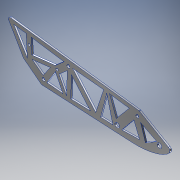
# Autodesk Inventor part: bracket1
Saved by Autodesk Inventor 2018.2 (Build 222227000, 227)
## iProperties
Created: 2018-03-05
Part Number: bracket1
Material: アルミニウム 6061
Document SubType Name: Modeling
Designer: ku_sk
Density: 2.7 g/cm^3
Appearance: アルミニウム - フラット
Mass: 349.891 g
Surface Area: 692.084 cm^2
Volume: 129.589 cm^3
Author: ku_sk
Autodesk Inventor part; units mm, degrees
ref_plane "YZ Plane" through (0, 0, 0) normal (1, 0, 0) x (0, 1, 0)
ref_plane "XZ Plane" through (0, 0, 0) normal (0, 1, 0) x (-1, 0, 0)
ref_plane "XY Plane" through (0, 0, 0) normal (0, 0, 1) x (1, 0, 0)
sketch "スケッチ2" plane through (0, 0, 0) normal (0, 1, 0) x (-1, 0, 0)
  arc A0 (320.7468, 34.8983) -> (392.1215, 71.6787) centre (243.1623, 273.099) ccw projected
  arc A1 (310.5095, 31.8959) -> (320.7468, 34.8983) centre (264.9264, 206.2785) ccw projected
  arc A2 (290.9118, 29.5172) -> (310.5095, 31.8959) centre (291.9468, 102.9093) ccw projected
  arc A3 (278.6891, 31.4878) -> (290.9118, 29.5172) centre (291.5128, 72.1352) ccw projected
  arc A4 (274.9831, 33.389) -> (278.6891, 31.4878) centre (282.4278, 43.3382) ccw projected
  arc A5 (275.4733, 39.2078) -> (274.9831, 33.389) centre (277.0456, 36.1453) ccw projected
  arc A6 (283.1253, 42.3274) -> (275.4733, 39.2078) centre (297.1464, -3.0086) ccw projected
  arc A7 (310.1184, 49.282) -> (283.1253, 42.3274) centre (369.3413, -236.446) ccw projected
  arc A8 (310.1184, 49.282) -> (326.9533, 52.7997) centre (-771.7798, 5269.0252) ccw projected
  arc A9 (326.9533, 52.7997) -> (357.98, 60.8795) centre (256.8539, 385.5961) ccw projected
  arc A10 (357.98, 60.8795) -> (391.1188, 73.3957) centre (268.9975, 346.6028) ccw projected
  arc A11 (392.1215, 71.6787) -> (391.1188, 73.3957) centre (391.5269, 72.4828) ccw projected
  circle A12 centre (287.1934, 37.1564) radius 3 projected
  circle A13 centre (359.7933, 56.2153) radius 3 projected
  arc A14 (100.5026, -29.4375) -> (303.8176, 17.6729) centre (68.6386, 570.3585) ccw projected
  arc A15 (74.9408, -30.0377) -> (100.5026, -29.4375) centre (77.5861, 401.9345) ccw projected
  arc A16 (28.1912, -23.4013) -> (74.9408, -30.0377) centre (76.0159, 145.5175) ccw projected
  arc A17 (1.2395, -11.312) -> (28.1912, -23.4013) centre (55.8939, 74.446) ccw projected
  arc A18 (-6.0217, -4.7376) -> (1.2395, -11.312) centre (16.9451, 13.3315) ccw projected
  arc A19 (-1.6159, 7.4897) -> (-6.0217, -4.7376) centre (0, 0) ccw projected
  arc A20 (17.9572, 9.9554) -> (-1.6159, 7.4897) centre (22.277, -103.2534) ccw projected
  arc A21 (84.7958, 9.311) -> (17.9572, 9.9554) centre (44.6377, -689.2581) ccw projected
  arc A22 (84.7958, 9.311) -> (126.0099, 7.0084) centre (819.0754, 12782.4716) ccw projected
  arc A23 (126.0099, 7.0084) -> (203.0122, 6.466) centre (170.258, 822.6468) ccw projected
  arc A24 (203.0122, 6.466) -> (303.8176, 17.6729) centre (174.1884, 724.7085) ccw projected
  circle A25 centre (20.0666, -1.5588) radius 5 projected
  circle A26 centre (130.4331, -10.1322) radius 5 projected
  line L0 (100.5026, -29.4375) -> (327.9026, -17.3569)
  line L1 (-3.831, 6.6355) -> (72.6844, 50.8117)
  line L2 (1137.2465, 0) -> (-1089.9509, 0) projected
  line L3 (72.6844, 50.8117) -> (483.7253, 102.9093)
  line L4 (327.9026, -17.3569) -> (483.7253, 102.9093)
  point P0 (0, 0)
  point P1 (371.2778, 57.8193)
  dimension "d7" = 30
  constraints: 8 end point, 2 point on circle, 2 tangent
  measures "d7" angle of L2 L1
extrude "押し出し3" add sketch "スケッチ2" along normal blind 4 contours A1 A2 A3 A4 A5 A6 A7 A8 A9 A10 A11 A0 | A15 A16 A17 A18 A19 L2 A25 A14 | A14 L2 L4 L0 | L2 A25 A19 A20 A21 A22 A23 A24 A14 | A14 A24 A23 A22 A21 A20 A19 L1 L3 L4 L2
sketch "スケッチ3" plane through (0, 4, 0) normal (0, 1, 0) x (1, 0, 0)
  line L0 (-483.7253, -102.9093) -> (-72.6844, -50.8117) projected
  line L1 (-327.9026, 17.3569) -> (-483.7253, -102.9093) projected
  line L2 (-483.7253, -102.9093) -> (-72.6844, -50.8117) projected
  line L3 (-418.3387, -94.6218) -> (-374.803, -18.8415)
  line L4 (-327.9026, 17.3569) -> (-483.7253, -102.9093) projected
  point P0 (0, 0)
  constraints: 2 end point, 2 point on line
extrude "押し出し4" cut sketch "スケッチ3" against normal through all
fillet "フィレット2" radius 5 4 edges at (-418.3387, 2, 94.6218) (-72.6844, 2, 50.8117) (-327.9026, 2, -17.3569) (-374.803, 2, 18.8415)
sketch "スケッチ4" plane through (0, 4, 0) normal (0, 1, 0) x (1, 0, 0)
  circle A0 centre (-77.5679, -36.3106) radius 4
  circle A1 centre (-322.4385, 2.626) radius 4
  circle A2 centre (-257.5679, -59.1248) radius 4
  line L0 (-71.8122, -50.3081) -> (3.831, -6.6355) projected
  line L1 (-408.3679, -93.358) -> (-73.6835, -50.9383) projected
  line L2 (-100.5026, 29.4375) -> (-326.3465, 17.4396) projected
  line L3 (-329.1362, 16.4048) -> (-374.0171, -18.2349) projected
  point P0 (0, 0)
  dimension "d15" = 15
  dimension "d16" = 15
  dimension "d17" = 8
  dimension "d18" = 15
  dimension "d19" = 8
  dimension "d20" = 180
  dimension "d21" = 8
  dimension "d22" = 15
  dimension "d23" = 15
  constraints: 3 centre point
  measures "d15" distance from line of L0 A0.centre
  measures "d16" distance from line of A0.centre L1
  measures "d17" diameter of A0
  measures "d18" distance from line of L1 A2.centre
  measures "d19" diameter of A2
  measures "d20" horizontal distance of A0.centre A2.centre
  measures "d21" diameter of A1
  measures "d22" distance from line of L2 A1.centre
  measures "d23" distance from line of L3 A1.centre
extrude "押し出し5" cut sketch "スケッチ4" against normal through all
sketch "スケッチ5" plane through (0, 0, 0) normal (0, -1, 0) x (1, 0, 0)
  line L0 (-399.8979, 82.3649) -> (-367.9521, 78.2557)
  line L1 (-367.9521, 78.2557) -> (-364.6383, 23.9082)
  line L2 (-364.6383, 23.9082) -> (-399.8979, 82.3649)
  line L3 (-355.0856, 76.6007) -> (-352.6658, 36.9174)
  line L4 (-352.6658, 36.9174) -> (-291.6076, 44.0321)
  line L5 (-291.6076, 44.0321) -> (-269.0016, 63.509)
  line L6 (-269.0016, 63.509) -> (-355.0856, 76.6007)
  line L7 (-352.0763, 27.2481) -> (-304.6777, 32.7712)
  line L8 (-304.6777, 32.7712) -> (-323.2812, 5.7482)
  line L9 (-323.2812, 5.7482) -> (-352.0763, 27.2481)
  line L10 (-291.4126, 29.994) -> (-271.7097, -9.6068)
  line L11 (-271.7097, -9.6068) -> (-313.7076, -5.8004)
  line L12 (-313.7076, -5.8004) -> (-291.4126, 29.994)
  line L13 (-282.0681, 29.2322) -> (-262.3081, -10.4835)
  line L14 (-262.3081, -10.4835) -> (-260.4868, 47.8263)
  line L15 (-260.4868, 47.8263) -> (-282.0681, 29.2322)
  line L16 (-249.6696, 44.1742) -> (-251.4069, -11.4469)
  line L17 (-251.4069, -11.4469) -> (-200.374, -13.041)
  line L18 (-200.374, -13.041) -> (-249.6696, 44.1742)
  line L19 (-246.2929, 60.0555) -> (-186.2732, -9.6068)
  line L20 (-186.2732, -9.6068) -> (-165.4814, 52.2118)
  line L21 (-165.4814, 52.2118) -> (-246.2929, 60.0555)
  line L22 (-150.4021, 50.7481) -> (-98.7306, 43.6255)
  line L23 (-150.4021, 50.7481) -> (-132.7161, 3.5142)
  line L24 (-132.7161, 3.5142) -> (-98.7306, 43.6255)
  line L25 (-173.5739, -13.8781) -> (-141.5591, -14.8781)
  line L26 (-141.5591, -14.8781) -> (-157.5665, 48.0655)
  line L27 (-157.5665, 48.0655) -> (-173.5739, -13.8781)
  line L28 (-86.7096, 23.5699) -> (-118.3577, -14.9798)
  line L29 (-118.3577, -14.9798) -> (-71.5255, -13.8781)
  line L30 (-71.5255, -13.8781) -> (-86.7096, 23.5699)
  line L31 (-69.1982, 26.078) -> (-56.4892, -13.5243)
  line L32 (-56.4892, -13.5243) -> (-26.7058, 4.295)
  line L33 (-26.7058, 4.295) -> (-69.1982, 26.078)
  point P0 (0, 0)
  constraints: 68 end point, 10 point on line, 5 parallel, 3 perpendicular
extrude "押し出し6" cut sketch "スケッチ5" against normal through all
sketch "スケッチ6" plane through (0, 0, 0) normal (0, -1, 0) x (1, 0, 0)
  circle A0 centre (-20.0666, -1.5588) radius 6
  circle A1 centre (-20.0666, -1.5588) radius 5 projected
  circle A2 centre (-130.4331, -10.1322) radius 6
  circle A3 centre (-130.4331, -10.1322) radius 5 projected
  point P0 (0, 0)
  dimension "d29" = 12
  dimension "d30" = 12
  constraints: 2 centre point, 2 concentric
  measures "d29" diameter of A0
  measures "d30" diameter of A2
extrude "押し出し7" cut sketch "スケッチ6" against normal through all
equation "\"d16\" = d15"
equation "\"d18\" = d16"
equation "\"d19\" = d17"
equation "\"d21\" = d19"
equation "\"d22\" = d18"
equation "\"d23\" = d22"
